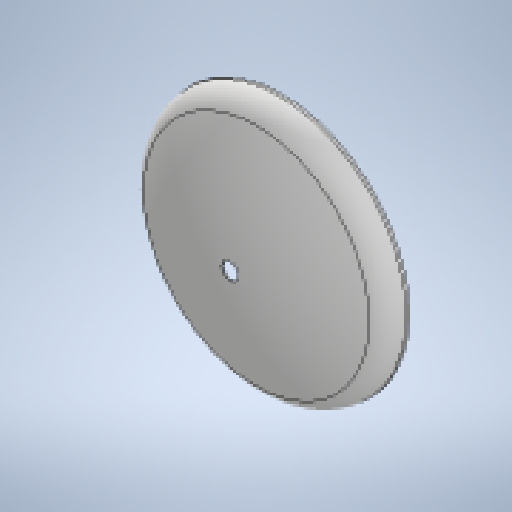
# Autodesk Inventor part: dished head
Saved by Autodesk Inventor 2025.1 (Build 291241020, 241B)
## iProperties
Created: 2024-12-11
Part Number: dished head
Material: Generic
Document SubType Name: Modeling
Designer: user
Density: 1 g/cm^3
Appearance: Default
Author: user
Autodesk Inventor part; units mm, degrees
ref_plane "YZ Plane" through (0, 0, 0) normal (1, 0, 0) x (0, 1, 0)
ref_plane "XZ Plane" through (0, 0, 0) normal (0, 1, 0) x (-1, 0, 0)
ref_plane "XY Plane" through (0, 0, 0) normal (0, 0, 1) x (1, 0, 0)
sketch "Sketch1" plane through (0, 0, 0) normal (0, 0, 1) x (1, 0, 0)
  line L0 (-666.6667, 586.2904) -> (666.6667, 586.2904) construction
  arc A0 (-666.6667, 586.2904) -> (0, 430) centre (0, 1930) ccw construction
  line L1 (-750, 720.6613) -> (750, 720.6613) construction
  arc A1 (-750, 720.6613) -> (-666.6667, 586.2904) centre (-600, 720.6613) ccw construction
  arc A2 (666.6667, 586.2904) -> (750, 720.6613) centre (600, 720.6613) ccw
  line L2 (-750, 720.6613) -> (-750, 738.6613)
  line L3 (750, 720.6613) -> (750, 738.6613)
  line L4 (-750, 738.6613) -> (0, 738.6613) construction
  line L5 (0, 738.6613) -> (0, 0)
  arc A3 (0, 430) -> (666.6667, 586.2904) centre (0, 1930) ccw
  line L6 (0, 738.6613) -> (750, 738.6613)
  dimension "d0" = 1500
  dimension "d1" = 150
  dimension "d2" = 18
  dimension "d3" = 1500
  dimension "d7_from_floor" = 430
  constraints: 14 end point, 8 point on circle, 4 centre point, 4 tangent, 3 horizontal, 3 vertical, 2 equal length, 1 equal radius, 1 point on line, 1 vertical alignment
  measures "d0" radius of A0
  measures "d1" radius of A1
  measures "d2" distance of L1.start L2.end
  measures "d3" distance of L1.start L1.end
  measures "d7_from_floor" distance of L5.end A0.end
revolve "Revolution1" add sketch "Sketch1" angle 360 about axis through (0, 738.6613, 0) along (0, -1, 0)
shell "Shell1" thickness 8 removed faces 1 at (313.1401, 738.6613, 219.0792)
sketch "Sketch2" plane through (0, 0, 0) normal (0, 1, 0) x (-1, 0, 0)
  circle A0 centre (0, 0) radius 50
  dimension "d10" = 100
  constraints: 1 centre point, 1 coincident
  measures "d10" diameter of A0
extrude "Extrusion1" cut sketch "Sketch2" along normal through all
equation "\"d0\" = d3"
equation "\"d3\" = MAIN_Filter_Diam"
equation "\"d10\" = MAIN_Outer_Tube_Diam"
equation "\"MAIN_Filter_Diam\" = 1500"
equation "\"MAIN_Outer_Tube_Diam\" = 100"
body "Solid1"
